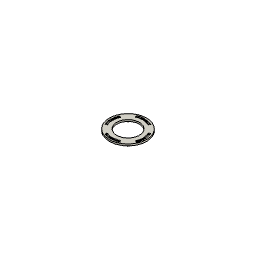
Speaker Lock Ring (Autodesk Fusion 360 design; units mm, degrees)
Autodesk Fusion 360 part; units mm, degrees
sketch "Sketch1" plane through (0, 0, 0) normal (0, 0, 1) x (1, 0, 0)
  circle A0 centre (0, 0) radius 46.2
  circle A1 centre (0, 0) radius 28
  circle A2 centre (0, 0) radius 42.55
  circle A3 centre (0, 0) radius 38.05
  circle A4 centre (0, 0) radius 41.75
  circle A5 centre (0, 0) radius 38.85
  line L0 (0, 0) -> (0, -38.05) construction
  line L1 (0, -38.05) -> (0, -42.55)
  line L2 (0, 0) -> (16.0806, -34.485) construction
  line L3 (0, 0) -> (38.3, 0) construction
  line L4 (16.0806, -34.485) -> (17.9824, -38.5634)
  line L5 (38.05, 0) -> (42.55, 0)
  line L6 (34.485, 16.0806) -> (38.5634, 17.9824)
  line L7 (0, 38.05) -> (0, 42.55)
  line L8 (-16.0806, 34.485) -> (-17.9824, 38.5634)
  line L9 (-38.05, 0) -> (-42.55, 0)
  line L10 (-34.485, -16.0806) -> (-38.5634, -17.9824)
  line L11 (0, 0) -> (-16.0806, -34.485) construction
  line L12 (-16.0806, -34.485) -> (-17.9824, -38.5634)
  line L13 (34.485, -16.0806) -> (38.5634, -17.9824)
  line L14 (16.0806, 34.485) -> (17.9824, 38.5634)
  line L15 (-34.485, 16.0806) -> (-38.5634, 17.9824)
  dimension "d105" = 92.4
  dimension "d106" = 56
  dimension "d107" = 85.1
  dimension "d108" = 76.1
  dimension "d109" = 83.5
  dimension "d110" = 77.7
  dimension "d111" = 38.05
  dimension "d113" = 25
  dimension "d115" = 360
  dimension "d117" = 25
  constraint coincident A0.centre A1.centre
  constraint concentric A0 A2
  constraint concentric A1 A3
  constraint concentric A1 A4
  constraint concentric A0 A5
  constraint vertical L0
  constraint vertical L1
  constraint coincident A2 L1.end
  constraint horizontal L3
  constraint coincident A3 L2.end
  constraint coincident A2 L4.end
  constraint parallel L2 L4
  constraint coincident A3 L11.end
  constraint coincident A2 L12.end
  constraint parallel L11 L12
  measures "d105" diameter of A0
  measures "d106" diameter of A1
  measures "d107" diameter of A2
  measures "d108" diameter of A3
  measures "d109" diameter of A4
  measures "d110" diameter of A5
  measures "d111" distance of A0.centre L0.end
  measures "d113" angle of L0 L2
  measures "d117" angle of L0 L11
extrude "Extrude1" add sketch "Sketch1" against normal blind 4 contours A0 | A2 A4 L5 L6 | A2 A4 L5 L13 | A2 A4 L6 L14 | A2 A4 L4 L13 | A4 A5 L5 L6 | A4 A5 L5 L13 | A2 A4 L7 L14 | A4 A5 L6 L14 | A2 A4 L1 L4 | A4 A5 L4 L13 | A3 A5 L5 L6 | A3 A5 L5 L13 | A2 A4 L7 L8 | A4 A5 L7 L14 | A3 A5 L6 L14 | A2 A4 L1 L12 | A4 A5 L1 L4 | A3 A5 L4 L13 | A3 | A2 A4 L8 L15 | A4 A5 L7 L8 | A3 A5 L7 L14 | A2 A4 L10 L12 | A4 A5 L1 L12 | A3 A5 L1 L4 | A2 A4 L9 L15 | A4 A5 L8 L15 | A3 A5 L7 L8 | A2 A4 L9 L10 | A4 A5 L10 L12 | A3 A5 L1 L12 | A4 A5 L9 L15 | A3 A5 L8 L15 | A4 A5 L9 L10 | A3 A5 L10 L12 | A3 A5 L9 L15 | A3 A5 L9 L10
extrude "Extrude2" cut sketch "Sketch1" against normal blind 2.5 contours A2 A4 L5 L6 | A2 A4 L5 L13 | A4 A5 L5 L6 | A4 A5 L5 L13 | A2 A4 L7 L14 | A2 A4 L1 L4 | A3 A5 L5 L6 | A3 A5 L5 L13 | A2 A4 L7 L8 | A4 A5 L7 L14 | A2 A4 L1 L12 | A4 A5 L1 L4 | A4 A5 L7 L8 | A3 A5 L7 L14 | A4 A5 L1 L12 | A3 A5 L1 L4 | A2 A4 L9 L15 | A3 A5 L7 L8 | A2 A4 L9 L10 | A3 A5 L1 L12 | A4 A5 L9 L15 | A4 A5 L9 L10 | A3 A5 L9 L15 | A3 A5 L9 L10
extrude "Extrude3" add sketch "Sketch1" against normal blind 1 contours A2 A4 L5 L13 | A2 A4 L7 L14 | A3 A5 L5 L13 | A2 A4 L1 L12 | A3 A5 L7 L14 | A2 A4 L9 L15 | A3 A5 L1 L12 | A3 A5 L9 L15
chamfer "Chamfer1" distance 0.5 angle 45 8 edges at (-40.7604, 9.0364, -1) (-37.9291, 8.4087, -1) (9.0364, 40.7604, -1) (8.4087, 37.9291, -1) (40.7604, -9.0364, -1) (37.9291, -8.4087, -1) (-9.0364, -40.7604, -1) (-8.4087, -37.9291, -1)
chamfer "Chamfer2" distance 0.5 distance2 15 4 edges at (-17.0315, -36.5242, -2.5) (-36.5242, 17.0315, -2.5) (17.0315, 36.5242, -2.5) (36.5242, -17.0315, -2.5) measured on face at (-16.8273, -36.0862, -1.8333) measured on face at (-36.9623, 17.2358, -1.8333) measured on face at (17.2358, 36.9623, -1.8333) measured on face at (36.0862, -16.8273, -1.8333)
fillet "Fillet1" radius 0.35 16 edges at (-41.2485, 9.1446, -1) (-40.7604, 9.0364, -0.5) (-37.441, 8.3005, -1) (-37.9291, 8.4087, -0.5) (9.0364, 40.7604, -0.5) (9.1446, 41.2485, -1) (8.4087, 37.9291, -0.5) (8.3005, 37.441, -1) (37.9291, -8.4087, -0.5) (37.441, -8.3005, -1) (40.7604, -9.0364, -0.5) (41.2485, -9.1446, -1) (-8.3005, -37.441, -1) (-8.4087, -37.9291, -0.5) (-9.0364, -40.7604, -0.5) (-9.1446, -41.2485, -1)
ref_plane "WorkPlane1" through (0, 0, -4) normal (0, 0, -1) x (-1, 0, 0)
sketch "Sketch2" plane through (0, 0, -4) normal (0, 0, -1) x (-1, 0, 0)
  line L0 (0, 0) -> (26.2337, -26.2337) construction
  line L1 (0, 0) -> (41, 0) construction
  circle A0 centre (26.2337, -26.2337) radius 2.5
  circle A1 centre (26.2337, 26.2337) radius 2.5
  circle A2 centre (-26.2337, 26.2337) radius 2.5
  circle A3 centre (-26.2337, -26.2337) radius 2.5
  dimension "d130" = 37.1
  dimension "d131" = 45
  dimension "d132" = 5
  dimension "d134" = 360
  constraint horizontal L1
  constraint coincident L0.start L1.start
  constraint coincident L0.end A0.centre
  measures "d130" distance of L0.start L0.end
  measures "d131" angle of L0 L1
  measures "d132" diameter of A0
extrude "Extrude4" add sketch "Sketch2" along normal blind 8
fillet "Fillet2" radius 2.5 4 edges at (-23.9028, -27.1377, -12) (-23.9028, 25.3296, -12) (28.5645, 25.3296, -12) (28.5645, -27.1377, -12)
ref_plane "WorkPlane2" through (0, 0, 1.75) normal (-0.707107, 0.707107, 0) x (0, 0, 1)
sketch "Sketch3" plane through (0, 0, 0) normal (-0.707107, 0.707107, 0) x (0, 0, 1)
  line L0 (0, 0) -> (-8, 0) construction
  circle A0 centre (-8, 0) radius 1
  dimension "d140" = 8
  dimension "d141" = 2
  constraint coincident L0.start origin
  constraint coincident L0.end A0.centre
  measures "d140" distance of L0.start L0.end
  measures "d141" diameter of A0
extrude "Extrude5" cut sketch "Sketch3" along normal through all and the other way through all
ref_plane "WorkPlane3" through (0, 0, 1.75) normal (0.707107, 0.707107, 0) x (0, 0, 1)
sketch "Sketch4" plane through (0, 0, 0) normal (0.707107, 0.707107, 0) x (0, 0, 1)
  line L0 (0, 0) -> (-8, 0) construction
  circle A0 centre (-8, 0) radius 1
  dimension "d144" = 8
  dimension "d145" = 2
  constraint coincident L0.start origin
  constraint coincident L0.end A0.centre
  measures "d144" distance of L0.start L0.end
  measures "d145" diameter of A0
extrude "Extrude6" cut sketch "Sketch4" along normal through all and the other way through all
equation "d105 = d1"
equation "d106 = d3"
equation "d107 = d4 + 0.5 mm"
equation "d108 = d5 - 0.5 mm"
equation "d109 = d14 + 0.5 mm"
equation "d110 = d15 - 0.5 mm"
equation "d111 = d108 / 2"
equation "d117 = d113"
equation "d118 = -4 mm"
equation "d130 = ( d105 - ( ( d105 - d106 ) / 2 ) ) / 2"
equation "d135 = 8 mm"
equation "d138 = d132 / 2"
equation "d140 = ( -d118 ) + ( d135 / 2 )"
equation "d144 = d140"
equation "d145 = d141"
equation "d1 = 92.4 mm"
equation "d3 = 56 mm"
equation "d4 = 84.6 mm"
equation "d5 = 76.6 mm"
equation "d14 = 83 mm"
equation "d15 = 78.2 mm"
